Autodesk Fusion 360 part; units mm, degrees
(part 4 of 4)
  constraint midpoint L87 L95.end
  constraint midpoint L93 L96.start
  constraint midpoint L83 L96.end
  constraint midpoint L92 L97.start
  constraint midpoint L79 L97.end
  constraint midpoint L91 L98.start
  constraint midpoint L75 L98.end
  constraint vertical L98
  constraint vertical L97
  constraint vertical L95
  constraint vertical L96
  constraint equal L97 L98
  constraint equal L96 L97
  constraint equal L95 L96
  constraint midpoint L78 L99.start
  constraint midpoint L76 L99.end
  constraint midpoint L82 L100.start
  constraint midpoint L80 L100.end
  constraint midpoint L86 L101.start
  constraint midpoint L84 L101.end
  constraint midpoint L90 L102.start
  constraint midpoint L88 L102.end
  constraint midpoint L99 P11
  constraint midpoint L100 P12
  constraint midpoint L101 P13
  constraint midpoint L102 P14
  constraint coincident L53 L103.start
  constraint coincident L51 L103.end
  constraint perpendicular L51 L103
  constraint coincident L103 L113.start
  constraint coincident L112 L113.end
  constraint perpendicular L112 L113
  constraint coincident L112 L115.start
  constraint coincident L103 L115.end
  constraint perpendicular L103 L115
  constraint equal L114 L116
  constraint coincident L103 L117.end
  constraint coincident L103 L118.end
  constraint coincident L103 L119.end
  constraint coincident L103 L120.end
  constraint equal L120 L121
  constraint equal L119 L120
  constraint equal L118 L119
  constraint equal L117 L118
  constraint coincident L112 L122.end
  constraint perpendicular L112 L122
  constraint coincident L112 L123.end
  constraint perpendicular L112 L123
  constraint coincident L112 L124.end
  constraint perpendicular L112 L124
  constraint perpendicular L52 L125
  constraint horizontal L126
  constraint vertical L127
  constraint horizontal L128
  constraint vertical L129
  constraint horizontal L130
  constraint vertical L131
  constraint horizontal L132
  constraint vertical L133
  constraint midpoint L128 P15
  constraint midpoint L132 P16
  constraint coincident L111 L134.start
  constraint coincident L122 L134.start
  constraint coincident L111 L134.end
  constraint coincident L123 L134.end
  constraint coincident L111 L135.start
  constraint coincident L124 L135.start
  constraint coincident L111 L135.end
  constraint coincident L125 L135.end
  constraint midpoint P16 L135
  constraint midpoint P15 L134
  constraint equal L126 L129
  constraint equal L130 L131
  constraint equal L129 L131
  constraint equal L78 L129
  constraint midpoint L127 L136.start
  constraint midpoint L129 L136.end
  constraint midpoint L131 L137.start
  constraint midpoint L133 L137.end
  constraint midpoint L136 L138.start
  constraint perpendicular L111 L138
  constraint midpoint L137 L139.start
  constraint perpendicular L137 L139
  constraint equal L138 L139
  constraint coincident L110 L140.start
  constraint coincident L124 L140.start
  constraint coincident L109 L140.end
  constraint coincident L123 L140.end
  constraint coincident L107 L141.start
  constraint coincident L124 L141.start
  constraint coincident L123 L141.end
  constraint parallel L140 L141
  constraint coincident L104 L142.end
  constraint coincident L124 L142.end
  constraint coincident L108 L143.start
  constraint coincident L113 L143.start
  constraint coincident L108 L143.end
  constraint coincident L122 L143.end
  constraint coincident L123 L144.end
  constraint coincident L108 L144.end
  constraint coincident L108 L145.end
  constraint coincident L124 L145.end
  constraint coincident L125 L146.end
  constraint coincident L108 L146.end
  constraint coincident L108 L147.end
  constraint coincident L115 L147.end
  constraint coincident L105 L148.start
  constraint coincident L113 L148.start
  constraint coincident L105 L148.end
  constraint coincident L122 L148.end
  constraint coincident L123 L149.end
  constraint coincident L105 L149.end
  constraint coincident L105 L150.end
  constraint coincident L124 L150.end
  constraint coincident L105 L151.end
  constraint coincident L125 L151.end
  constraint coincident L105 L152.end
  constraint coincident L115 L152.end
  constraint horizontal L153
  constraint vertical L154
  constraint horizontal L155
  constraint vertical L156
  constraint horizontal L157
  constraint vertical L158
  constraint horizontal L159
  constraint vertical L160
  constraint horizontal L161
  constraint vertical L162
  constraint horizontal L163
  constraint vertical L164
  constraint horizontal L165
  constraint vertical L166
  constraint horizontal L167
  constraint vertical L168
  constraint equal L61 L161
  constraint equal L161 L164
  constraint equal L161 L165
  constraint equal L165 L168
  constraint equal L61 L153
  constraint equal L153 L154
  constraint equal L153 L157
  constraint equal L157 L158
  constraint midpoint L149 L161
  constraint midpoint L151 L165
  constraint midpoint L144 L153
  constraint midpoint L146 L157
  constraint midpoint L164 L169.start
  constraint midpoint L162 L169.end
  constraint midpoint L168 L170.start
  constraint midpoint L166 L170.end
  constraint midpoint L160 L171.start
  constraint midpoint L158 L171.end
  constraint midpoint L156 L172.start
  constraint midpoint L154 L172.end
  constraint midpoint L172 L173.start
  constraint perpendicular L153 L173
  constraint midpoint L171 L174.start
  constraint perpendicular L171 L174
  constraint midpoint L169 L175.start
  constraint perpendicular L161 L175
  constraint midpoint L170 L176.start
  constraint perpendicular L105 L176
  constraint equal L138 L173
  constraint equal L138 L175
  constraint equal L173 L174
  constraint equal L175 L176
  constraint horizontal L177
  constraint vertical L178
  constraint horizontal L179
  constraint vertical L180
  constraint horizontal L181
  constraint vertical L182
  constraint horizontal L183
  constraint vertical L184
  constraint horizontal L185
  constraint vertical L186
  constraint horizontal L187
  constraint vertical L188
  constraint horizontal L189
  constraint vertical L190
  constraint horizontal L191
  constraint vertical L192
  constraint horizontal L193
  constraint vertical L194
  constraint horizontal L195
  constraint vertical L196
  constraint horizontal L197
  constraint vertical L198
  constraint horizontal L199
  constraint vertical L200
  constraint parallel L201 L202
  constraint midpoint L148 L206
  constraint midpoint L150 L205
  constraint midpoint L152 L204
  constraint midpoint L147 L203
  constraint midpoint L145 L202
  constraint midpoint L143 L201
  constraint equal L153 L178
  constraint equal L178 L179
  constraint equal L153 L182
  constraint equal L153 L186
  constraint equal L186 L187
  measures "d377" distance of L13.start L16.end
  measures "d379" distance of L24 L26.end
  measures "d380" distance of L33.start L33.end
  measures "d381" distance of L30.end L31.end
  measures "d382" distance of L29.start L31.end
  measures "d385" distance of L35.end L36.end
  measures "d386" distance of L34.end L35.end
  measures "d387" distance of L29 L38
  measures "d388" distance of L34 L38
  measures "d389" distance of L30 L41
  measures "d390" distance of L39.end L40.end
  measures "d391" distance of L38.end L39.end
  measures "d393" vertical distance of L36.end P1
  measures "d400" diameter of A58
  measures "d402" distance of L37 L41
  measures "d403" horizontal distance of L35.end P1
  measures "d409" distance of L51.end L52.end
  measures "d410" distance of L50.start L52.end
  measures "d411" distance of L33.end L54.end
  measures "d412" distance of L35.end L57.end
  measures "d413" distance of L61.start L61.end
  measures "d414" distance of L55 L62
  measures "d415" vertical distance of L98.start L98.end
  measures "d420" distance of L112.start L113.end
  measures "d421" distance of L56 L103
  measures "d422" distance of L138.start L138.end
sketch "oled_screen_proto" plane through (0, 0, 0) normal (1, 0, 0) x (0, 0, -1)
  line L0 (7.25, 194.3) -> (78.25, 194.3)
  line L1 (7.25, 151.3) -> (7.25, 194.3)
  line L2 (78.25, 151.3) -> (7.25, 151.3)
  line L3 (78.25, 194.3) -> (78.25, 151.3)
  line L4 (76.35, 192.4) -> (76.35, 153.2)
  line L5 (76.35, 153.2) -> (9.15, 153.2)
  line L6 (74.05, 152.7) -> (11.95, 152.7)
  line L7 (74.05, 191.5) -> (74.05, 152.7)
  line L8 (11.95, 152.7) -> (11.95, 191.5)
  line L9 (9.15, 153.2) -> (9.15, 192.4)
  line L10 (9.15, 192.4) -> (76.35, 192.4)
  line L11 (11.95, 191.5) -> (74.05, 191.5)
  line L12 (71.5, 160) -> (71.5, 189.5)
  line L13 (14.5, 189.5) -> (14.5, 160)
  line L14 (71.5, 189.5) -> (14.5, 189.5)
  line L15 (14.5, 160) -> (71.5, 160)
  circle A0 centre (76.75, 165.18) radius 0.5
  circle A1 centre (76.75, 167.72) radius 0.5
  circle A2 centre (76.75, 170.26) radius 0.5
  circle A3 centre (76.75, 172.8) radius 0.5
  circle A4 centre (76.75, 175.34) radius 0.5
  circle A5 centre (76.75, 177.88) radius 0.5
  circle A6 centre (76.75, 180.42) radius 0.5
  point P0 (76.75, 180.42)
  point P1 (76.75, 177.88)
  point P2 (76.75, 175.34)
  point P3 (76.75, 172.8)
  point P4 (76.75, 170.26)
  point P5 (76.75, 167.72)
  point P6 (76.75, 165.18)
  dimension "d401" = 1
  constraint coincident P6 A0.centre
  constraint coincident P5 A1.centre
  constraint coincident P4 A2.centre
  constraint coincident P3 A3.centre
  constraint coincident P2 A4.centre
  constraint coincident P1 A5.centre
  constraint coincident P0 A6.centre
  constraint equal A5 A6
  constraint equal A4 A5
  constraint equal A3 A4
  constraint equal A2 A3
  constraint equal A1 A2
  constraint equal A0 A1
  measures "d401" diameter of A0
hidden bodies 1 2 3 4 5 6 7 8 9 10 11 12 13 14
equation "d21 = 6.5 mm - 2.5 mm"
equation "d46 = d45"
equation "d115 = 20.5 mm - 3 mm"
equation "d116 = 52 mm + 6 mm"
equation "d133 = 5.35 mm + 0.5 mm"
equation "d190 = ( ( 8 + 0.3 ) / 2 ) * 1 mm"
equation "d200 = 3 mm + 0.5 mm"
equation "d264 = ( ( 8 + 0.3 ) / 2 ) * 1 mm"
equation "d271 = ( ( 8 + 0.3 ) / 2 ) * 1 mm"
equation "d278 = ( ( 8 + 0.3 ) / 2 ) * 1 mm"
equation "d308 = ( 5.35 / 2 ) * 1 mm"
equation "d309 = d308"
equation "d310 = d309"
equation "d311 = d309"
equation "d312 = d311"
equation "d415 = d414"
named bodies: "switch_board", "switch_board_back_m3_spacer", "switch_board_front_m5_spacer", "switch_board_left_m5_spacer", "switch_board_right_m5_spacer", "audio_amp_spacer", "left_side_support", "right_side_support", "left_side_panel", "right_side_panel", "internal_nut_test", "layer_0_rpi_support", "layer_0", "layer_1"
